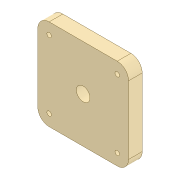
# Autodesk Inventor part: corpo_01b
Saved by Autodesk Inventor 2020 (Build 240168000, 168)
## iProperties
Created: 2022-07-20
Part Number: corpo_01b
Material: Genérico
Document SubType Name: Modeling
Designer: gabri
Density: 1 g/cm^3
Appearance: Bege
Author: gabri
Autodesk Inventor part; units mm, degrees
ref_plane "YZ Plane" through (0, 0, 0) normal (1, 0, 0) x (0, 1, 0)
ref_plane "XZ Plane" through (0, 0, 0) normal (0, 1, 0) x (-1, 0, 0)
ref_plane "Plano de trabalho1" through (0, 0, 0) normal (0, 0, 1) x (1, 0, 0)
sketch "Esboço1" plane through (0, 0, 0) normal (0, 0, 1) x (1, 0, 0)
  arc A0 (-40, -30) -> (-30, -40) centre (-30, -30) ccw
  line L0 (30, -40) -> (-30, -40)
  arc A1 (30, -40) -> (40, -30) centre (30, -30) ccw
  line L1 (40, 30) -> (40, -30)
  arc A2 (40, 30) -> (30, 40) centre (30, 30) ccw
  line L2 (-30, 40) -> (30, 40)
  arc A3 (-30, 40) -> (-40, 30) centre (-30, 30) ccw
  line L3 (-40, -30) -> (-40, 30)
  circle A4 centre (0, 0) radius 5
  circle A5 centre (0, 0) radius 6
  circle A6 centre (30, 30) radius 2
  circle A7 centre (30, -30) radius 2
  circle A8 centre (-30, -30) radius 2
  circle A9 centre (-30, 30) radius 2
  point P0 (0, 0)
  dimension "d0" = 12
  dimension "d3" = 4
  dimension "d4" = 4
  dimension "d5" = 4
  dimension "d6" = 4
  dimension "d7" = 80
  constraints: 10 centre point, 8 end point, 8 point on circle, 5 coincident
  measures "d0" diameter of A5
  measures "d3" diameter of A6
  measures "d4" diameter of A7
  measures "d5" diameter of A8
  measures "d6" diameter of A9
  measures "d7" distance between parallel lines of L0 L2
extrude "Extrusão1" add sketch "Esboço1" along normal blind 12 contours L3 A3 L2 A2 L1 A1 L0 A0
equation "\"d3\" = d6"
equation "\"d4\" = d6"
equation "\"d5\" = d6"
